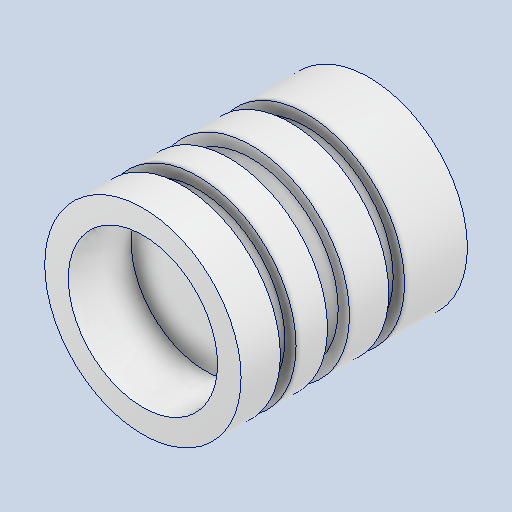
# Autodesk Inventor part: felga
Saved by Autodesk Inventor 2023 (Build 270158000, 158)
## iProperties
Created: 2022-12-08
Part Number: felga
Material: Aluminum 6061
Document SubType Name: Modeling
Designer: Kamil
Density: 2.7 g/cm^3
Appearance: Aluminum - Flat
Mass: 20.7607 g
Surface Area: 50.8115 cm^2
Volume: 7.68915 cm^3
Author: Kamil
Autodesk Inventor part; units mm, degrees
ref_plane "YZ Plane" through (0, 0, 0) normal (1, 0, 0) x (0, 1, 0)
sketch "Sketch1" plane through (0, 0, 0) normal (0, 0, 1) x (1, 0, 0)
  circle A0 centre (0, 0) radius 0.5 projected
  circle A1 centre (0, 0) radius 8.1639
  point P0 (0, 0)
  constraints: 1 centre point, 1 coincident
extrude "Extrusion1" add sketch "Sketch1" along normal blind 9.8
ref_plane "Work Plane1" through (0, 0, -10) normal (0, 0, 1) x (1, 0, 0)
sketch "Sketch2" plane through (0, 0, -10) normal (0, 0, 1) x (1, 0, 0)
  line L0 (5, 5) -> (-5, 5) projected
  arc A0 (-5, 5) -> (-6, 4) centre (-5, 4) ccw projected
  line L1 (-6, 4) -> (-6, -4) projected
  arc A1 (-6, -4) -> (-5, -5) centre (-5, -4) ccw projected
  line L2 (-5, -5) -> (5, -5) projected
  arc A2 (5, -5) -> (6, -4) centre (5, -4) ccw projected
  line L3 (6, -4) -> (6, 4) projected
  arc A3 (6, 4) -> (5, 5) centre (5, 4) ccw projected
  circle A4 centre (3.5, 2.5) radius 1.75 projected
  circle A5 centre (-3.5, -2.5) radius 1.75 projected
  circle A6 centre (4.5, 0) radius 0.625 projected
  circle A7 centre (-4.5, 0) radius 0.625 projected
  circle A8 centre (0, 0) radius 2 projected
  line L4 (0, 0) -> (5.8769, -4.8974)
  line L5 (5.8769, -4.8974) -> (7.0292, -5.8577)
  circle A9 centre (0, 0) radius 9.15
  circle A10 centre (0, 0) radius 8.1639 projected
  circle A11 centre (0, 0) radius 13.1
  line L6 (3.0438, -10.097) -> (-9.0477, 9.4736)
  line L7 (-6.9043, 6.0044) -> (-9.0477, 9.4736)
  line L8 (3.0438, -10.097) -> (-5, 4)
  line L9 (-5, 4) -> (-4.2491, 2.684)
  point P0 (0, 0)
  dimension "d3" = 26.2
  dimension "d2" = 1.5
  dimension "d4" = 18.3
  constraints: 12 end point, 3 point on line, 2 coincident, 2 point on circle, 1 centre point, 1 collinear, 3 other
  measures "d2" distance of L4.end L5.end
  measures "d4" diameter of A9
extrude "Extrusion2" add sketch "Sketch2" against normal blind 9 contours A9 L8 L6 | A11
sketch "Sketch3" plane through (0, 0, -10) normal (0, 0, 1) x (1, 0, 0)
  arc A0 (0.8877, 1.2091) -> (1.103, -1.0166) centre (0, 0) ccw projected
  line L0 (0.8877, 1.2091) -> (1.103, -1.0166) projected
  circle A1 centre (0, 0) radius 13.1 projected
  circle A2 centre (0, 0) radius 9.15 projected
  circle A3 centre (0, 0) radius 8.1639 projected
  circle A4 centre (0, 0) radius 0.5 projected
  point P0 (0, 0)
extrude "Extrusion3" add sketch "Sketch3" along normal up to surface (19.8 mm away) contours A1 | A2 | A3
sketch "Sketch4" plane through (0, 0, 9.8) normal (0, 0, 1) x (1, 0, 0)
  circle A0 centre (0, 0) radius 13.1 projected
  circle A1 centre (0, 0) radius 0.5 projected
  point P0 (0, 0)
extrude "Extrusion4" add sketch "Sketch4" against normal blind 10 contours A1
sketch "Sketch5" plane through (0, 0, 9.8) normal (0, 0, 1) x (1, 0, 0)
  circle A0 centre (0, 0) radius 13.1 projected
  point P0 (0, 0)
extrude "Extrusion5" add sketch "Sketch5" against normal up to surface (9.8 mm away)
sketch "Sketch6" plane through (0, 0, -0.2) normal (0, 0, -1) x (-1, 0, 0)
  circle A0 centre (0, 0) radius 0.5 projected
  point P0 (0, 0)
extrude "Extrusion6" cut sketch "Sketch6" against normal up to surface (0.2 mm away)
sketch "Sketch8" plane through (0, 0, 9.8) normal (0, 0, 1) x (1, 0, 0)
  circle A0 centre (0, 0) radius 13.1 projected
  point P0 (0, 0)
extrude "Extrusion7" cut sketch "Sketch8" against normal blind 3
sketch "Sketch10" plane through (0, 0, -19) normal (0, 0, -1) x (-1, 0, 0)
  circle A0 centre (0, 0) radius 13.1 projected
  circle A1 centre (0, 0) radius 9.15 projected
  circle A2 centre (0, 0) radius 12.5
  line L0 (-12.5, 0) -> (-9.15, 0)
  circle A3 centre (0, 0) radius 9.15 projected
  line L1 (-9.15, 0) -> (-10.825, 0)
  circle A4 centre (0, 0) radius 10.825
  point P0 (0, 0)
  dimension "d18" = 25
  constraints: 4 end point, 2 coincident, 2 horizontal alignment, 2 point on circle, 1 horizontal, 1 midpoint, 4 other
extrude "Extrusion8" cut sketch "Sketch10" against normal up to surface (9 mm away)
extrude "Extrusion9" cut sketch "Sketch10" against normal through all contours A0
sketch "Sketch11" plane through (0, 0, -19) normal (0, 0, -1) x (-1, 0, 0)
  circle A0 centre (0, 0) radius 10.825 projected
  line L0 (-0.8877, 1.2091) -> (-1.103, -1.0166) projected
  arc A1 (-1.103, -1.0166) -> (-0.8877, 1.2091) centre (0, 0) ccw projected
  circle A2 centre (0, 0) radius 10.825 projected
  circle A3 centre (0, 0) radius 12.5 projected
  line L1 (-12.5, 0) -> (-9.5, 0)
  circle A4 centre (0, 0) radius 9.5
  point P0 (0, 0)
  dimension "d23" = 3
  constraints: 2 end point, 2 horizontal alignment, 1 coincident, 1 horizontal, 3 other
  measures "d23" distance of L1.start L1.end
extrude "Extrusion10" add sketch "Sketch11" against normal up to surface (9 mm away) contours A0
sketch "Sketch12" plane through (0, 0, 6.8) normal (0, 0, 1) x (1, 0, 0)
  circle A0 centre (0, 0) radius 12.5 projected
  circle A1 centre (0, 0) radius 9.5 projected
  line L0 (0.8877, 1.2091) -> (1.103, -1.0166) projected
  arc A2 (0.8877, 1.2091) -> (1.103, -1.0166) centre (0, 0) ccw projected
  point P0 (0, 0)
extrude "Extrusion11" cut sketch "Sketch12" against normal blind 8 contours A1 | L0 A2
sketch "Sketch13" plane through (0, 0, -1.2) normal (0, 0, 1) x (1, 0, 0)
  line L0 (1.103, -1.0166) -> (0.8877, 1.2091) projected
  arc A0 (0.8877, 1.2091) -> (1.103, -1.0166) centre (0, 0) ccw projected
  circle A1 centre (0, 0) radius 9.5 projected
  circle A2 centre (0, 0) radius 11.0657
  circle A3 centre (0, 0) radius 9.5 projected
  circle A4 centre (0, 0) radius 12.5 projected
  point P0 (0, 0)
  constraints: 1 centre point, 1 coincident
extrude "Extrusion12" cut sketch "Sketch13" against normal up to surface (8.8 mm away) contours A4
sketch "Sketch14" plane through (0, 0, -10) normal (0, 0, 1) x (1, 0, 0)
  circle A0 centre (0, 0) radius 11.0657 projected
  circle A1 centre (0, 0) radius 12.5 projected
  point P0 (0, 0)
extrude "Extrusion13" add sketch "Sketch14" along normal blind 3
sketch "Sketch15" plane through (0, 0, -1.2) normal (0, 0, -1) x (-1, 0, 0)
  circle A0 centre (0, 0) radius 12.5 projected
  circle A1 centre (0, 0) radius 11.0657 projected
  point P0 (0, 0)
extrude "Extrusion14" add sketch "Sketch15" along normal blind 3
ref_plane "Work Plane2" through (0, 0, -14) normal (0, 0, -1) x (-1, 0, 0)
ref_plane "Work Plane3" through (0, 0, 1.8) normal (0, 0, 1) x (1, 0, 0)
sketch "Sketch16" plane through (0, 0, -14) normal (0, 0, -1) x (-1, 0, 0)
  circle A0 centre (0, 0) radius 12.5 projected
  circle A1 centre (0, 0) radius 11.0657 projected
  point P0 (0, 0)
extrude "Extrusion15" cut sketch "Sketch16" against normal blind 2
sketch "Sketch17" plane through (0, 0, 1.8) normal (0, 0, 1) x (1, 0, 0)
  circle A0 centre (0, 0) radius 12.5 projected
  circle A1 centre (0, 0) radius 11.0657 projected
  point P0 (0, 0)
extrude "Extrusion16" cut sketch "Sketch17" against normal blind 2
sketch "Sketch18" plane through (0, 0, -19) normal (0, 0, -1) x (-1, 0, 0)
  circle A0 centre (0, 0) radius 9.5 projected
  circle A1 centre (0, 0) radius 12.5 projected
  point P0 (0, 0)
extrude "Extrusion17" add sketch "Sketch18" along normal blind 2
sketch "Sketch19" plane through (0, 0, -21) normal (0, 0, -1) x (-1, 0, 0)
  circle A0 centre (0, 0) radius 12.5 projected
  circle A1 centre (0, 0) radius 9.5 projected
  point P0 (0, 0)
extrude "Extrusion18" add sketch "Sketch19" along normal blind 1
body "Solid1"
